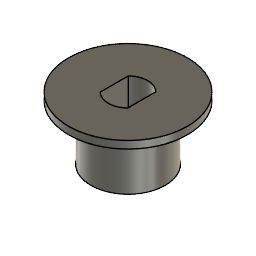
motor_shaft_slot (Autodesk Fusion 360 design; units mm, degrees)
part number: 2026-04-08-09-22-26-219
Autodesk Fusion 360 part; units mm, degrees
note: some values were not read from the file. Set by a fixed rule: which sketch regions a step uses.
sketch "Sketch1" plane through (0, 0, 0) normal (0, 0, 1) x (1, 0, 0)
  circle A0 centre (0, 0) radius 2.65
  circle A1 centre (0, 0) radius 5
  line L0 (0, 0.6) -> (0, -0.4) construction
  line L1 (0, 0) -> (-2.65, 0)
  line L2 (-1.85, 1.8974) -> (-1.85, -1.8974)
  line L3 (1.85, 1.8974) -> (1.85, -1.8974)
  dimension "d2" = 10
  dimension "d10" = 1.85
  dimension "d11" = 5.3
  constraint coincident A0.centre A1.centre
  constraint concentric A0 A1
  constraint vertical L0
  constraint coincident A0 L1.end
  constraint perpendicular L0 L1
  constraint perpendicular L1 L2
  constraint coincident A0 L2.start
  constraint coincident A0 L2.end
  constraint symmetric L0 L2.start L3.start
  constraint symmetric L0 L2.end L3.end
  measures "d2" diameter of A1
  measures "d10" distance of L0 L2
  measures "d11" diameter of A0
extrude "Extrude1" add sketch "Sketch1" against normal blind 8.4 contours A0 L3 | A0 L1 L2 | A0 L1 L2 | A1
sketch "Sketch2" plane through (0, 0, 0) normal (0, 0, 1) x (1, 0, 0)
  circle A0 centre (0, 0) radius 8
  circle A1 centre (0, 0) radius 5
  dimension "d5" = 16
  dimension "d6" = 10
  constraint coincident A0.centre A1.centre
  measures "d5" diameter of A0
  measures "d6" diameter of A1
extrude "Extrude2" add sketch "Sketch2" against normal blind 1
